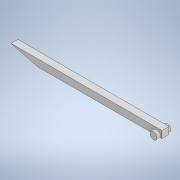
# Autodesk Inventor part: Crossbow entry
Saved by Autodesk Inventor 2021 (Build 250183000, 183)
## iProperties
Created: 2020-07-07
Part Number: Crossbow entry
Material: Generic
Document SubType Name: Modeling
Designer: saipr
Density: 1 g/cm^3
Appearance: Default
Author: saipr
Autodesk Inventor part; units mm, degrees
ref_plane "YZ Plane" through (0, 0, 0) normal (1, 0, 0) x (0, 1, 0)
ref_plane "XZ Plane" through (0, 0, 0) normal (0, 1, 0) x (-1, 0, 0)
ref_plane "XY Plane" through (0, 0, 0) normal (0, 0, 1) x (1, 0, 0)
sketch "Sketch1" plane through (0, 0, 0) normal (0, 0, 1) x (1, 0, 0)
  line L0 (0, 0) -> (55.1478, 0)
  line L1 (55.1478, 0) -> (55.1478, 2.54)
  line L2 (55.1478, 2.54) -> (0, 2.54)
  line L3 (0, 2.54) -> (0, 0)
  circle A0 centre (53.34, 0.635) radius 1.27
  point P0 (52.2401, 0)
  point P1 (54.4399, 0)
  dimension "d1" = 2.54
  constraints: 8 end point, 2 parallel, 1 centre point, 1 horizontal, 1 perpendicular
  measures "d1" distance of L1.end L0.end
extrude "Extrusion1" add sketch "Sketch1" along normal blind 2.54 contours L3 L2 L1 L0 A0
extrude "Extrusion2" add sketch "Sketch1" along normal blind 3.81 contours A0 L0 | L0 A0
extrude "Extrusion3" add sketch "Sketch1" against normal blind 1.27 contours A0 L0 | L0 A0
sketch "Sketch2" plane through (0, 0, 2.54) normal (0, 0, 1) x (1, 0, 0)
  line L0 (55.1478, 2.54) -> (0, 2.54) projected
  line L1 (0, 2.54) -> (9.8291, 0)
  line L2 (0, 0) -> (52.2401, 0) projected
  line L3 (0, 2.54) -> (0, 0)
  line L4 (9.8291, 0) -> (0, 0)
  constraints: 6 end point, 1 perpendicular, 1 point on line
extrude "Extrusion4" cut sketch "Sketch2" against normal blind 2.54
body "Solid1"
